Autodesk Fusion 360 part; units mm, degrees
note: some values were not read from the file. Set by a fixed rule: which sketch regions a step uses.
(part 2 of 5)
  spline S303 degree 3 poles (-4.641177, -45.308539) (-4.430839, -45.084511) (-4.24446, -44.841814) (-4.08204, -44.58107) knots 0 0 0 0 1 1 1 1
  spline S304 degree 3 poles (-4.08204, -44.58107) (-3.919308, -44.320326) (-3.783958, -44.045892) (-3.675366, -43.758389) knots 0 0 0 0 1 1 1 1
  spline S305 degree 3 poles (-3.675366, -43.758389) (-3.566775, -43.470575) (-3.487431, -43.175293) (-3.437025, -42.871922) knots 0 0 0 0 1 1 1 1
  spline S306 degree 3 poles (-3.437025, -42.871922) (-3.344302, -42.440045) (-3.20584, -42.023415) (-3.02164, -41.622031) knots 0 0 0 0 1 1 1 1
  spline S307 degree 3 poles (-3.02164, -41.622031) (-2.837439, -41.220647) (-2.611855, -40.844155) (-2.344576, -40.492244) knots 0 0 0 0 1 1 1 1
  line L5 (-2.344576, -40.492244) -> (-2.0885, -40.180472)
  spline S308 degree 3 poles (-2.0885, -40.180472) (-2.072631, -40.162736) (-2.058941, -40.143756) (-2.047117, -40.12322) knots 0 0 0 0 1 1 1 1
  spline S309 degree 3 poles (-2.047117, -40.12322) (-2.035293, -40.102684) (-2.025647, -40.081215) (-2.01818, -40.058812) knots 0 0 0 0 1 1 1 1
  spline S310 degree 3 poles (-2.01818, -40.058812) (-2.010712, -40.036409) (-2.005423, -40.013695) (-2.002622, -39.990048) knots 0 0 0 0 1 1 1 1
  spline S311 degree 3 poles (-2.002622, -39.990048) (-1.999822, -39.966711) (-1.9992, -39.943064) (-2.001067, -39.919728) knots 0 0 0 0 1 1 1 1
  spline S312 degree 3 poles (-2.001067, -39.919728) (-2.002934, -39.89608) (-2.006978, -39.872744) (-2.013513, -39.85003) knots 0 0 0 0 1 1 1 1
  spline S313 degree 3 poles (-2.013513, -39.85003) (-2.020047, -39.827316) (-2.028759, -39.805535) (-2.039649, -39.784688) knots 0 0 0 0 1 1 1 1
  spline S314 degree 3 poles (-2.039649, -39.784688) (-2.050539, -39.76353) (-2.063608, -39.743928) (-2.078232, -39.72557) knots 0 0 0 0 1 1 1 1
  spline S315 degree 3 poles (-2.078232, -39.72557) (-2.093167, -39.707212) (-2.109658, -39.690721) (-2.128016, -39.675475) knots 0 0 0 0 1 1 1 1
  spline S316 degree 3 poles (-2.128016, -39.675475) (-2.146063, -39.660539) (-2.165665, -39.647471) (-2.186512, -39.63627) knots 0 0 0 0 1 1 1 1
  spline S317 degree 3 poles (-2.186512, -39.63627) (-2.207359, -39.625379) (-2.22914, -39.616356) (-2.251854, -39.609822) knots 0 0 0 0 1 1 1 1
  spline S318 degree 3 poles (-2.251854, -39.609822) (-2.274568, -39.602979) (-2.297593, -39.598621) (-2.320929, -39.596754) knots 0 0 0 0 1 1 1 1
  spline S319 degree 3 poles (-2.320929, -39.596754) (-2.344576, -39.594578) (-2.367913, -39.594889) (-2.39156, -39.597685) knots 0 0 0 0 1 1 1 1
  spline S320 degree 3 poles (-2.39156, -39.597685) (-2.414896, -39.600169) (-2.437922, -39.605466) (-2.460324, -39.61262) knots 0 0 0 0 1 1 1 1
  spline S321 degree 3 poles (-2.460324, -39.61262) (-2.482727, -39.620083) (-2.504197, -39.629422) (-2.524732, -39.641246) knots 0 0 0 0 1 1 1 1
  spline S322 degree 3 poles (-2.524732, -39.641246) (-2.545268, -39.652758) (-2.56456, -39.666449) (-2.582295, -39.682006) knots 0 0 0 0 1 1 1 1
  spline S323 degree 3 poles (-2.582295, -39.682006) (-2.600031, -39.697564) (-2.616211, -39.714677) (-2.630524, -39.733346) knots 0 0 0 0 1 1 1 1
  line L6 (-2.630524, -39.733346) -> (-2.899669, -40.06161)
  spline S324 degree 3 poles (-2.899669, -40.06161) (-3.204285, -40.460193) (-3.460673, -40.888025) (-3.668832, -41.344482) knots 0 0 0 0 1 1 1 1
  spline S325 degree 3 poles (-3.668832, -41.344482) (-3.87668, -41.801251) (-4.031322, -42.275444) (-4.132447, -42.767061) knots 0 0 0 0 1 1 1 1
  spline S326 degree 3 poles (-12.220487, -38.608227) (-12.202752, -39.475091) (-12.270582, -40.335111) (-12.423046, -41.188596) knots 0 0 0 0 1 1 1 1
  line L7 (-12.423046, -41.188596) -> (-12.452605, -41.369997)
  spline S327 degree 3 poles (-12.452605, -41.369997) (-12.545017, -41.884328) (-12.549062, -42.399282) (-12.46474, -42.914547) knots 0 0 0 0 1 1 1 1
  spline S328 degree 3 poles (-12.46474, -42.914547) (-12.460694, -42.93695) (-12.454472, -42.95873) (-12.446071, -42.979888) knots 0 0 0 0 1 1 1 1
  spline S329 degree 3 poles (-12.446071, -42.979888) (-12.43767, -43.001047) (-12.427091, -43.021271) (-12.414956, -43.040563) knots 0 0 0 0 1 1 1 1
  spline S330 degree 3 poles (-12.414956, -43.040563) (-12.40251, -43.059543) (-12.388507, -43.077278) (-12.372951, -43.093769) knots 0 0 0 0 1 1 1 1
  spline S331 degree 3 poles (-12.372951, -43.093769) (-12.357082, -43.11026) (-12.339969, -43.124884) (-12.3213, -43.137953) knots 0 0 0 0 1 1 1 1
  spline S332 degree 3 poles (-12.3213, -43.137953) (-12.302631, -43.151021) (-12.28303, -43.162222) (-12.262181, -43.171557) knots 0 0 0 0 1 1 1 1
  spline S333 degree 3 poles (-12.262181, -43.171557) (-12.241334, -43.180891) (-12.219865, -43.188048) (-12.197773, -43.193026) knots 0 0 0 0 1 1 1 1
  spline S334 degree 3 poles (-12.197773, -43.193026) (-12.175682, -43.198005) (-12.153279, -43.201116) (-12.130565, -43.201738) knots 0 0 0 0 1 1 1 1
  spline S335 degree 3 poles (-12.130565, -43.201738) (-12.107851, -43.202375) (-12.085137, -43.201102) (-12.062734, -43.197382) knots 0 0 0 0 1 1 1 1
  spline S336 degree 3 poles (-12.062734, -43.197382) (-12.040331, -43.193646) (-12.01824, -43.187737) (-11.997081, -43.179958) knots 0 0 0 0 1 1 1 1
  spline S337 degree 3 poles (-11.997081, -43.179958) (-11.975612, -43.171868) (-11.955387, -43.161911) (-11.936096, -43.150087) knots 0 0 0 0 1 1 1 1
  spline S338 degree 3 poles (-11.936096, -43.150087) (-11.916493, -43.138264) (-11.898447, -43.124573) (-11.881645, -43.109327) knots 0 0 0 0 1 1 1 1
  spline S339 degree 3 poles (-11.881645, -43.109327) (-11.864842, -43.093769) (-11.849907, -43.076967) (-11.836217, -43.058609) knots 0 0 0 0 1 1 1 1
  spline S340 degree 3 poles (-11.836217, -43.058609) (-11.822837, -43.040251) (-11.811325, -43.02096) (-11.801368, -43.000113) knots 0 0 0 0 1 1 1 1
  spline S341 degree 3 poles (-11.801368, -43.000113) (-11.791722, -42.979577) (-11.784255, -42.958419) (-11.778654, -42.936327) knots 0 0 0 0 1 1 1 1
  spline S342 degree 3 poles (-11.778654, -42.936327) (-11.773054, -42.914236) (-11.76963, -42.891833) (-11.768386, -42.869119) knots 0 0 0 0 1 1 1 1
  spline S343 degree 3 poles (-11.768386, -42.869119) (-11.767144, -42.846405) (-11.768067, -42.823691) (-11.77119, -42.800977) knots 0 0 0 0 1 1 1 1
  spline S344 degree 3 poles (-11.77119, -42.800977) (-11.842754, -42.361633) (-11.839021, -41.9226) (-11.759677, -41.4845) knots 0 0 0 0 1 1 1 1
  line L8 (-11.759677, -41.4845) -> (-11.730429, -41.297188)
  spline S345 degree 3 poles (-11.730429, -41.297188) (-11.569563, -40.38894) (-11.500178, -39.473847) (-11.522581, -38.551909) knots 0 0 0 0 1 1 1 1
  line L9 (-11.522581, -38.551909) -> (-11.685312, -37.17538)
  spline S346 degree 3 poles (-11.685312, -37.17538) (-11.68998, -37.138042) (-11.700248, -37.102259) (-11.716116, -37.068033) knots 0 0 0 0 1 1 1 1
  spline S347 degree 3 poles (-11.716116, -37.068033) (-11.732296, -37.033806) (-11.753143, -37.003002) (-11.778969, -36.975621) knots 0 0 0 0 1 1 1 1
  spline S348 degree 3 poles (-11.778969, -36.975621) (-11.805105, -36.94824) (-11.834665, -36.925526) (-11.867646, -36.90779) knots 0 0 0 0 1 1 1 1
  spline S349 degree 3 poles (-11.867646, -36.90779) (-11.90094, -36.889744) (-11.936099, -36.877609) (-11.973126, -36.871075) knots 0 0 0 0 1 1 1 1
  spline S350 degree 3 poles (-11.973126, -36.871075) (-12.000196, -36.866096) (-12.027578, -36.864543) (-12.054959, -36.866096) knots 0 0 0 0 1 1 1 1
  spline S351 degree 3 poles (-12.054959, -36.866096) (-12.08234, -36.867338) (-12.10941, -36.872317) (-12.135547, -36.880098) knots 0 0 0 0 1 1 1 1
  spline S352 degree 3 poles (-12.135547, -36.880098) (-12.161995, -36.887879) (-12.187198, -36.898767) (-12.210845, -36.912458) knots 0 0 0 0 1 1 1 1
  spline S353 degree 3 poles (-12.210845, -36.912458) (-12.234804, -36.926148) (-12.256583, -36.942639) (-12.276809, -36.961308) knots 0 0 0 0 1 1 1 1
  spline S354 degree 3 poles (-12.276809, -36.961308) (-12.296723, -36.980288) (-12.314147, -37.001136) (-12.329393, -37.024161) knots 0 0 0 0 1 1 1 1
  spline S355 degree 3 poles (-12.329393, -37.024161) (-12.344329, -37.047186) (-12.356775, -37.071767) (-12.366109, -37.097592) knots 0 0 0 0 1 1 1 1
  spline S356 degree 3 poles (-12.366109, -37.097592) (-12.375444, -37.123418) (-12.381667, -37.150176) (-12.384778, -37.177558) knots 0 0 0 0 1 1 1 1
  spline S357 degree 3 poles (-12.384778, -37.177558) (-12.387892, -37.204939) (-12.387892, -37.23232) (-12.38446, -37.25939) knots 0 0 0 0 1 1 1 1
  line L10 (-12.38446, -37.25939) -> (-12.220487, -38.608227)
  spline S358 degree 3 poles (-10.950372, -36.928949) (-10.779861, -38.496835) (-10.819377, -40.059743) (-11.068609, -41.61705) knots 0 0 0 0 1 1 1 1
  spline S359 degree 3 poles (-11.068609, -41.61705) (-11.085722, -41.719418) (-11.097857, -41.822409) (-11.105013, -41.925711) knots 0 0 0 0 1 1 1 1
  spline S360 degree 3 poles (-11.105013, -41.925711) (-11.112166, -42.029324) (-11.114348, -42.132937) (-11.111234, -42.23655) knots 0 0 0 0 1 1 1 1
  spline S361 degree 3 poles (-11.111234, -42.23655) (-11.10812, -42.340474) (-11.100033, -42.443776) (-11.086964, -42.546456) knots 0 0 0 0 1 1 1 1
  spline S362 degree 3 poles (-11.086964, -42.546456) (-11.073896, -42.649447) (-11.055538, -42.751504) (-11.032513, -42.852628) knots 0 0 0 0 1 1 1 1
  spline S363 degree 3 poles (-11.032513, -42.852628) (-11.009488, -42.953752) (-10.981173, -43.053631) (-10.948191, -43.151954) knots 0 0 0 0 1 1 1 1
  spline S364 degree 3 poles (-10.948191, -43.151954) (-10.915209, -43.250278) (-10.87756, -43.346734) (-10.835244, -43.441324) knots 0 0 0 0 1 1 1 1
  spline S365 degree 3 poles (-10.835244, -43.441324) (-10.792927, -43.535914) (-10.745944, -43.628325) (-10.694293, -43.718248) knots 0 0 0 0 1 1 1 1
  spline S366 degree 3 poles (-10.694293, -43.718248) (-10.642953, -43.808482) (-10.586946, -43.895604) (-10.526894, -43.980236) knots 0 0 0 0 1 1 1 1
  spline S367 degree 3 poles (-10.526894, -43.980236) (-10.466842, -44.064558) (-10.403056, -44.14608) (-10.334914, -44.224178) knots 0 0 0 0 1 1 1 1
  spline S368 degree 3 poles (-10.334914, -44.224178) (-10.266773, -44.302588) (-10.195208, -44.377264) (-10.11991, -44.448206) knots 0 0 0 0 1 1 1 1
  spline S369 degree 3 poles (-10.11991, -44.448206) (-10.044301, -44.51946) (-9.96558, -44.586668) (-9.883747, -44.650143) knots 0 0 0 0 1 1 1 1
  spline S370 degree 3 poles (-9.883747, -44.650143) (-9.801604, -44.713618) (-9.716971, -44.772736) (-9.628915, -44.82781) knots 0 0 0 0 1 1 1 1
  spline S371 degree 3 poles (-9.628915, -44.82781) (-9.541171, -44.882883) (-9.450937, -44.933601) (-9.358215, -44.979651) knots 0 0 0 0 1 1 1 1
  spline S372 degree 3 poles (-9.358215, -44.979651) (-9.265492, -45.026013) (-9.170591, -45.067396) (-9.073823, -45.104422) knots 0 0 0 0 1 1 1 1
  spline S373 degree 3 poles (-9.073823, -45.104422) (-8.977055, -45.141138) (-8.878421, -45.173187) (-8.778542, -45.200257) knots 0 0 0 0 1 1 1 1
  spline S374 degree 3 poles (-8.778542, -45.200257) (-8.678662, -45.227327) (-8.577538, -45.24973) (-8.47517, -45.266843) knots 0 0 0 0 1 1 1 1
  spline S375 degree 3 poles (-8.47517, -45.266843) (-8.373113, -45.283956) (-8.270433, -45.296091) (-8.16682, -45.303247) knots 0 0 0 0 1 1 1 1
  spline S376 degree 3 poles (-8.16682, -45.303247) (-8.063518, -45.310402) (-7.960216, -45.312582) (-7.856603, -45.309468) knots 0 0 0 0 1 1 1 1
  spline S377 degree 3 poles (-7.856603, -45.309468) (-7.75299, -45.306354) (-7.649688, -45.298267) (-7.547009, -45.284887) knots 0 0 0 0 1 1 1 1
  spline S378 degree 3 poles (-7.547009, -45.284887) (-7.444329, -45.271819) (-7.342272, -45.253461) (-7.24146, -45.230125) knots 0 0 0 0 1 1 1 1
  spline S379 degree 3 poles (-7.24146, -45.230125) (-7.140336, -45.2071) (-7.040768, -45.178785) (-6.942444, -45.145803) knots 0 0 0 0 1 1 1 1
  spline S380 degree 3 poles (-6.942444, -45.145803) (-6.844121, -45.112821) (-6.747975, -45.074861) (-6.653386, -45.032544) knots 0 0 0 0 1 1 1 1
  spline S381 degree 3 poles (-6.653386, -45.032544) (-6.558796, -44.989917) (-6.466695, -44.942933) (-6.376772, -44.891282) knots 0 0 0 0 1 1 1 1
  spline S382 degree 3 poles (-6.376772, -44.891282) (-6.28685, -44.839631) (-6.199417, -44.783624) (-6.115095, -44.723572) knots 0 0 0 0 1 1 1 1
  spline S383 degree 3 poles (-6.115095, -44.723572) (-6.030773, -44.66352) (-5.949252, -44.599112) (-5.871153, -44.53097) knots 0 0 0 0 1 1 1 1
  spline S384 degree 3 poles (-5.871153, -44.53097) (-5.793055, -44.462828) (-5.718378, -44.390952) (-5.647436, -44.315654) knots 0 0 0 0 1 1 1 1
  spline S385 degree 3 poles (-5.647436, -44.315654) (-5.576183, -44.240045) (-5.508974, -44.161323) (-5.4455, -44.07918) knots 0 0 0 0 1 1 1 1
  spline S386 degree 3 poles (-5.4455, -44.07918) (-5.382336, -43.997036) (-5.322906, -43.911781) (-5.268144, -43.824037) knots 0 0 0 0 1 1 1 1
  spline S387 degree 3 poles (-5.268144, -43.824037) (-5.21307, -43.735981) (-5.162353, -43.645747) (-5.116303, -43.552714) knots 0 0 0 0 1 1 1 1
  spline S388 degree 3 poles (-5.116303, -43.552714) (-5.069941, -43.45968) (-5.028558, -43.364779) (-4.991843, -43.2677) knots 0 0 0 0 1 1 1 1
  spline S389 degree 3 poles (-4.991843, -43.2677) (-4.954816, -43.170932) (-4.922767, -43.072297) (-4.895697, -42.972107) knots 0 0 0 0 1 1 1 1
  spline S390 degree 3 poles (-4.895697, -42.972107) (-4.868627, -42.871917) (-4.846224, -42.770793) (-4.829111, -42.668424) knots 0 0 0 0 1 1 1 1
  spline S391 degree 3 poles (-4.829111, -42.668424) (-4.7423, -42.276997) (-4.627486, -41.893971) (-4.484668, -41.519346) knots 0 0 0 0 1 1 1 1
  spline S392 degree 3 poles (-4.484668, -41.519346) (-4.34185, -41.144721) (-4.172584, -40.782543) (-3.976559, -40.43281) knots 0 0 0 0 1 1 1 1
  spline S393 degree 3 poles (-3.976559, -40.43281) (-3.780846, -40.083077) (-3.560551, -39.749524) (-3.315676, -39.43215) knots 0 0 0 0 1 1 1 1
  spline S394 degree 3 poles (-3.315676, -39.43215) (-3.070801, -39.114777) (-2.804456, -38.817006) (-2.51602, -38.538838) knots 0 0 0 0 1 1 1 1
  spline S395 degree 3 poles (-2.51602, -38.538838) (-2.499529, -38.522347) (-2.485216, -38.504611) (-2.472459, -38.48532) knots 0 0 0 0 1 1 1 1
  spline S396 degree 3 poles (-2.472459, -38.48532) (-2.45939, -38.466029) (-2.448811, -38.445804) (-2.440099, -38.424334) knots 0 0 0 0 1 1 1 1
  spline S397 degree 3 poles (-2.440099, -38.424334) (-2.431076, -38.402865) (-2.424541, -38.381085) (-2.420185, -38.358371) knots 0 0 0 0 1 1 1 1
  spline S398 degree 3 poles (-2.420185, -38.358371) (-2.415518, -38.335657) (-2.41334, -38.312632) (-2.413651, -38.289606) knots 0 0 0 0 1 1 1 1
  spline S399 degree 3 poles (-2.413651, -38.289606) (-2.413651, -38.266581) (-2.415829, -38.243556) (-2.420497, -38.220842) knots 0 0 0 0 1 1 1 1
  spline S400 degree 3 poles (-2.420497, -38.220842) (-2.424853, -38.198128) (-2.431698, -38.176348) (-2.440721, -38.154878) knots 0 0 0 0 1 1 1 1
  spline S401 degree 3 poles (-2.440721, -38.154878) (-2.449434, -38.13372) (-2.460324, -38.113184) (-2.473081, -38.094204) knots 0 0 0 0 1 1 1 1
  spline S402 degree 3 poles (-2.473081, -38.094204) (-2.486149, -38.074913) (-2.500773, -38.057177) (-2.516953, -38.040997) knots 0 0 0 0 1 1 1 1
  spline S403 degree 3 poles (-2.516953, -38.040997) (-2.533444, -38.024506) (-2.55118, -38.010193) (-2.570471, -37.997125) knots 0 0 0 0 1 1 1 1
  spline S404 degree 3 poles (-2.570471, -37.997125) (-2.589762, -37.984368) (-2.609987, -37.973789) (-2.631145, -37.964766) knots 0 0 0 0 1 1 1 1
  spline S405 degree 3 poles (-2.631145, -37.964766) (-2.652615, -37.956053) (-2.674706, -37.949519) (-2.69742, -37.945163) knots 0 0 0 0 1 1 1 1
  spline S406 degree 3 poles (-2.69742, -37.945163) (-2.719823, -37.940496) (-2.742848, -37.93832) (-2.765873, -37.93832) knots 0 0 0 0 1 1 1 1
  spline S407 degree 3 poles (-2.765873, -37.93832) (-2.788898, -37.938639) (-2.811924, -37.940805) (-2.834638, -37.945474) knots 0 0 0 0 1 1 1 1
  spline S408 degree 3 poles (-2.834638, -37.945474) (-2.85704, -37.94983) (-2.879132, -37.956676) (-2.90029, -37.965699) knots 0 0 0 0 1 1 1 1
  spline S409 degree 3 poles (-2.90029, -37.965699) (-2.92176, -37.974411) (-2.941984, -37.985301) (-2.961276, -37.99837) knots 0 0 0 0 1 1 1 1
  spline S410 degree 3 poles (-2.961276, -37.99837) (-2.980256, -38.011127) (-2.997991, -38.025751) (-3.014171, -38.042242) knots 0 0 0 0 1 1 1 1
  spline S411 degree 3 poles (-3.014171, -38.042242) (-3.329367, -38.345613) (-3.620292, -38.670766) (-3.887259, -39.017698) knots 0 0 0 0 1 1 1 1
  spline S412 degree 3 poles (-3.887259, -39.017698) (-4.153915, -39.36432) (-4.393812, -39.728988) (-4.606327, -40.111391) knots 0 0 0 0 1 1 1 1
  spline S413 degree 3 poles (-4.606327, -40.111391) (-4.818843, -40.494106) (-5.00211, -40.890201) (-5.155819, -41.299985) knots 0 0 0 0 1 1 1 1
  spline S414 degree 3 poles (-5.155819, -41.299985) (-5.309216, -41.70977) (-5.431809, -42.128579) (-5.523287, -42.556721) knots 0 0 0 0 1 1 1 1
  spline S415 degree 3 poles (-5.523287, -42.556721) (-5.536666, -42.636376) (-5.55409, -42.715097) (-5.575249, -42.792885) knots 0 0 0 0 1 1 1 1
  spline S416 degree 3 poles (-5.575249, -42.792885) (-5.596407, -42.870983) (-5.621611, -42.947526) (-5.650237, -43.022825) knots 0 0 0 0 1 1 1 1
  spline S417 degree 3 poles (-5.650237, -43.022825) (-5.678862, -43.098434) (-5.711221, -43.172177) (-5.747315, -43.244364) knots 0 0 0 0 1 1 1 1
  spline S418 degree 3 poles (-5.747315, -43.244364) (-5.783408, -43.316862) (-5.822614, -43.38687) (-5.865552, -43.455323) knots 0 0 0 0 1 1 1 1
  spline S419 degree 3 poles (-5.865552, -43.455323) (-5.908491, -43.523777) (-5.954541, -43.58974) (-6.004014, -43.653837) knots 0 0 0 0 1 1 1 1
  spline S420 degree 3 poles (-6.004014, -43.653837) (-6.053487, -43.717623) (-6.105761, -43.77892) (-6.161145, -43.837416) knots 0 0 0 0 1 1 1 1
  spline S421 degree 3 poles (-6.161145, -43.837416) (-6.216529, -43.896223) (-6.274715, -43.951919) (-6.335389, -44.005126) knots 0 0 0 0 1 1 1 1
  spline S422 degree 3 poles (-6.335389, -44.005126) (-6.396374, -44.058022) (-6.459538, -44.107806) (-6.525502, -44.154478) knots 0 0 0 0 1 1 1 1
  spline S423 degree 3 poles (-6.525502, -44.154478) (-6.591154, -44.201151) (-6.658985, -44.244712) (-6.728993, -44.28485) knots 0 0 0 0 1 1 1 1
  spline S424 degree 3 poles (-6.728993, -44.28485) (-6.799002, -44.324989) (-6.870878, -44.361393) (-6.94431, -44.394375) knots 0 0 0 0 1 1 1 1
  spline S425 degree 3 poles (-6.94431, -44.394375) (-7.018053, -44.427357) (-7.09304, -44.456605) (-7.169582, -44.482431) knots 0 0 0 0 1 1 1 1
  spline S426 degree 3 poles (-7.169582, -44.482431) (-7.245815, -44.507945) (-7.323602, -44.529725) (-7.402011, -44.547772) knots 0 0 0 0 1 1 1 1
  spline S427 degree 3 poles (-7.402011, -44.547772) (-7.480732, -44.565819) (-7.560076, -44.579821) (-7.640041, -44.590089) knots 0 0 0 0 1 1 1 1
  spline S428 degree 3 poles (-7.640041, -44.590089) (-7.720007, -44.600045) (-7.800284, -44.606268) (-7.880872, -44.608758) knots 0 0 0 0 1 1 1 1
  spline S429 degree 3 poles (-7.880872, -44.608758) (-7.96146, -44.610933) (-8.041736, -44.609394) (-8.122324, -44.603779) knots 0 0 0 0 1 1 1 1
  spline S430 degree 3 poles (-8.122324, -44.603779) (-8.202601, -44.59787) (-8.282567, -44.588533) (-8.362221, -44.574842) knots 0 0 0 0 1 1 1 1
  spline S431 degree 3 poles (-8.362221, -44.574842) (-8.441565, -44.561463) (-8.520286, -44.544038) (-8.598073, -44.52288) knots 0 0 0 0 1 1 1 1
  spline S432 degree 3 poles (-8.598073, -44.52288) (-8.675861, -44.501722) (-8.752404, -44.476519) (-8.827702, -44.447893) knots 0 0 0 0 1 1 1 1
  spline S433 degree 3 poles (-8.827702, -44.447893) (-8.903, -44.418956) (-8.976743, -44.386596) (-9.048619, -44.350503) knots 0 0 0 0 1 1 1 1
  spline S434 degree 3 poles (-9.048619, -44.350503) (-9.120806, -44.314409) (-9.191126, -44.275205) (-9.259267, -44.232266) knots 0 0 0 0 1 1 1 1
  spline S435 degree 3 poles (-9.259267, -44.232266) (-9.327409, -44.189327) (-9.393373, -44.142966) (-9.457159, -44.093493) knots 0 0 0 0 1 1 1 1
  spline S436 degree 3 poles (-9.457159, -44.093493) (-9.520945, -44.04402) (-9.58193, -43.991747) (-9.640738, -43.936362) knots 0 0 0 0 1 1 1 1
  spline S437 degree 3 poles (-9.640738, -43.936362) (-9.699234, -43.880666) (-9.75493, -43.822481) (-9.807825, -43.761495) knots 0 0 0 0 1 1 1 1
  spline S438 degree 3 poles (-9.807825, -43.761495) (-9.86041, -43.700821) (-9.910194, -43.637346) (-9.956866, -43.571383) knots 0 0 0 0 1 1 1 1
  spline S439 degree 3 poles (-9.956866, -43.571383) (-10.003539, -43.50573) (-10.046789, -43.437588) (-10.086616, -43.367579) knots 0 0 0 0 1 1 1 1
  spline S440 degree 3 poles (-10.086616, -43.367579) (-10.126754, -43.29757) (-10.163159, -43.225695) (-10.19583, -43.151952) knots 0 0 0 0 1 1 1 1
  spline S441 degree 3 poles (-10.19583, -43.151952) (-10.228812, -43.078209) (-10.25806, -43.003222) (-10.283574, -42.926368) knots 0 0 0 0 1 1 1 1
  spline S442 degree 3 poles (-10.283574, -42.926368) (-10.309089, -42.849825) (-10.330869, -42.772349) (-10.348605, -42.693628) knots 0 0 0 0 1 1 1 1
  spline S443 degree 3 poles (-10.348605, -42.693628) (-10.366651, -42.614907) (-10.380653, -42.535563) (-10.39061, -42.455286) knots 0 0 0 0 1 1 1 1
  spline S444 degree 3 poles (-10.39061, -42.455286) (-10.400878, -42.375321) (-10.40679, -42.295044) (-10.408968, -42.214145) knots 0 0 0 0 1 1 1 1
  spline S445 degree 3 poles (-10.408968, -42.214145) (-10.411142, -42.133557) (-10.409605, -42.052969) (-10.403989, -41.972381) knots 0 0 0 0 1 1 1 1
  spline S446 degree 3 poles (-10.403989, -41.972381) (-10.398079, -41.891793) (-10.388432, -41.811828) (-10.375052, -41.732173) knots 0 0 0 0 1 1 1 1
  spline S447 degree 3 poles (-10.375052, -41.732173) (-10.115553, -40.106413) (-10.075104, -38.475363) (-10.254326, -36.838713) knots 0 0 0 0 1 1 1 1
  line L11 (-10.254326, -36.838713) -> (-10.390299, -35.753109)
  spline S448 degree 3 poles (-10.390299, -35.753109) (-10.394966, -35.715771) (-10.405545, -35.6803) (-10.421414, -35.646385) knots 0 0 0 0 1 1 1 1
  spline S449 degree 3 poles (-10.421414, -35.646385) (-10.437594, -35.612158) (-10.458441, -35.581665) (-10.484266, -35.554284) knots 0 0 0 0 1 1 1 1
  spline S450 degree 3 poles (-10.484266, -35.554284) (-10.510092, -35.527214) (-10.539651, -35.5045) (-10.572633, -35.486765) knots 0 0 0 0 1 1 1 1
  spline S451 degree 3 poles (-10.572633, -35.486765) (-10.605615, -35.469029) (-10.640775, -35.456894) (-10.677802, -35.45036) knots 0 0 0 0 1 1 1 1
  spline S452 degree 3 poles (-10.677802, -35.45036) (-10.71265, -35.443828) (-10.747499, -35.442897) (-10.78297, -35.447246) knots 0 0 0 0 1 1 1 1
  spline S453 degree 3 poles (-10.78297, -35.447246) (-10.805684, -35.450049) (-10.828087, -35.455027) (-10.850179, -35.462492) knots 0 0 0 0 1 1 1 1
  spline S454 degree 3 poles (-10.850179, -35.462492) (-10.871959, -35.469646) (-10.893118, -35.479295) (-10.913031, -35.490496) knots 0 0 0 0 1 1 1 1
  spline S455 degree 3 poles (-10.913031, -35.490496) (-10.932945, -35.502009) (-10.951925, -35.515388) (-10.969349, -35.530323) knots 0 0 0 0 1 1 1 1
  spline S456 degree 3 poles (-10.969349, -35.530323) (-10.986774, -35.54557) (-11.002643, -35.562372) (-11.016644, -35.580418) knots 0 0 0 0 1 1 1 1
  spline S457 degree 3 poles (-11.016644, -35.580418) (-11.030957, -35.598776) (-11.043092, -35.618379) (-11.05336, -35.638915) knots 0 0 0 0 1 1 1 1
  spline S458 degree 3 poles (-11.05336, -35.638915) (-11.063939, -35.659762) (-11.072029, -35.681231) (-11.078252, -35.703323) knots 0 0 0 0 1 1 1 1
  spline S459 degree 3 poles (-11.078252, -35.703323) (-11.084163, -35.725726) (-11.088209, -35.74844) (-11.089765, -35.771465) knots 0 0 0 0 1 1 1 1
  spline S460 degree 3 poles (-11.089765, -35.771465) (-11.091318, -35.79449) (-11.091007, -35.817515) (-11.0879, -35.84054) knots 0 0 0 0 1 1 1 1
  line L12 (-11.0879, -35.84054) -> (-10.950372, -36.928949)
  spline S461 degree 3 poles (-9.684301, -41.864103) (-9.694258, -41.921044) (-9.701414, -41.977984) (-9.705459, -42.035547) knots 0 0 0 0 1 1 1 1
  spline S462 degree 3 poles (-9.705459, -42.035547) (-9.709817, -42.09311) (-9.71137, -42.150673) (-9.710127, -42.208236) knots 0 0 0 0 1 1 1 1
  spline S463 degree 3 poles (-9.710127, -42.208236) (-9.708573, -42.265798) (-9.704527, -42.323361) (-9.69737, -42.380302) knots 0 0 0 0 1 1 1 1
  spline S464 degree 3 poles (-9.69737, -42.380302) (-9.690527, -42.437553) (-9.680567, -42.494494) (-9.668121, -42.550501) knots 0 0 0 0 1 1 1 1
  spline S465 degree 3 poles (-9.668121, -42.550501) (-9.655675, -42.606819) (-9.640118, -42.662204) (-9.622382, -42.716966) knots 0 0 0 0 1 1 1 1
  spline S466 degree 3 poles (-9.622382, -42.716966) (-9.604336, -42.771729) (-9.583489, -42.825558) (-9.560152, -42.878142) knots 0 0 0 0 1 1 1 1
  spline S467 degree 3 poles (-9.560152, -42.878142) (-9.537127, -42.931038) (-9.511302, -42.982377) (-9.482987, -43.032473) knots 0 0 0 0 1 1 1 1
  spline S468 degree 3 poles (-9.482987, -43.032473) (-9.454672, -43.082568) (-9.423868, -43.131418) (-9.390575, -43.178402) knots 0 0 0 0 1 1 1 1
  spline S469 degree 3 poles (-9.390575, -43.178402) (-9.357593, -43.225697) (-9.322433, -43.271125) (-9.284784, -43.314686) knots 0 0 0 0 1 1 1 1
  spline S470 degree 3 poles (-9.284784, -43.314686) (-9.247135, -43.358247) (-9.207619, -43.399941) (-9.165925, -43.439768) knots 0 0 0 0 1 1 1 1
  spline S471 degree 3 poles (-9.165925, -43.439768) (-9.124231, -43.479596) (-9.08067, -43.517245) (-9.035242, -43.552716) knots 0 0 0 0 1 1 1 1
  spline S472 degree 3 poles (-9.035242, -43.552716) (-8.990125, -43.588187) (-8.943141, -43.62148) (-8.894291, -43.652284) knots 0 0 0 0 1 1 1 1
  spline S473 degree 3 poles (-8.894291, -43.652284) (-8.845751, -43.683088) (-8.795967, -43.711403) (-8.744316, -43.737228) knots 0 0 0 0 1 1 1 1
  spline S474 degree 3 poles (-8.744316, -43.737228) (-8.692976, -43.763365) (-8.640392, -43.786701) (-8.586874, -43.807548) knots 0 0 0 0 1 1 1 1
  spline S475 degree 3 poles (-8.586874, -43.807548) (-8.533045, -43.828084) (-8.478594, -43.846131) (-8.423209, -43.861688) knots 0 0 0 0 1 1 1 1
  spline S476 degree 3 poles (-8.423209, -43.861688) (-8.367514, -43.876935) (-8.311506, -43.889692) (-8.254877, -43.899649) knots 0 0 0 0 1 1 1 1
  spline S477 degree 3 poles (-8.254877, -43.899649) (-8.198247, -43.909294) (-8.140996, -43.916451) (-8.083744, -43.920807) knots 0 0 0 0 1 1 1 1
  spline S478 degree 3 poles (-8.083744, -43.920807) (-8.026181, -43.925163) (-7.968619, -43.926407) (-7.911056, -43.925163) knots 0 0 0 0 1 1 1 1
  spline S479 degree 3 poles (-7.911056, -43.925163) (-7.853804, -43.92361) (-7.796241, -43.919562) (-7.739301, -43.912406) knots 0 0 0 0 1 1 1 1
  spline S480 degree 3 poles (-7.739301, -43.912406) (-7.682049, -43.905244) (-7.62542, -43.895604) (-7.569102, -43.882846) knots 0 0 0 0 1 1 1 1
  spline S481 degree 3 poles (-7.569102, -43.882846) (-7.513095, -43.8704) (-7.45771, -43.855154) (-7.402947, -43.837107) knots 0 0 0 0 1 1 1 1
  spline S482 degree 3 poles (-7.402947, -43.837107) (-7.348185, -43.818749) (-7.294668, -43.798214) (-7.242083, -43.774877) knots 0 0 0 0 1 1 1 1
  spline S483 degree 3 poles (-7.242083, -43.774877) (-7.189187, -43.751541) (-7.137847, -43.725716) (-7.087752, -43.697401) knots 0 0 0 0 1 1 1 1
  spline S484 degree 3 poles (-7.087752, -43.697401) (-7.037657, -43.668775) (-6.989117, -43.637971) (-6.942134, -43.604989) knots 0 0 0 0 1 1 1 1
  spline S485 degree 3 poles (-6.942134, -43.604989) (-6.894839, -43.571696) (-6.849723, -43.536225) (-6.805851, -43.498576) knots 0 0 0 0 1 1 1 1
  spline S486 degree 3 poles (-6.805851, -43.498576) (-6.762289, -43.460927) (-6.720595, -43.421411) (-6.681079, -43.379716) knots 0 0 0 0 1 1 1 1
  spline S487 degree 3 poles (-6.681079, -43.379716) (-6.641252, -43.338022) (-6.603603, -43.294461) (-6.568132, -43.249033) knots 0 0 0 0 1 1 1 1
  spline S488 degree 3 poles (-6.568132, -43.249033) (-6.532661, -43.203605) (-6.499679, -43.15631) (-6.468564, -43.107771) knots 0 0 0 0 1 1 1 1
  spline S489 degree 3 poles (-6.468564, -43.107771) (-6.43776, -43.05892) (-6.409446, -43.009136) (-6.38362, -42.957485) knots 0 0 0 0 1 1 1 1
  spline S490 degree 3 poles (-6.38362, -42.957485) (-6.357795, -42.906146) (-6.334147, -42.853561) (-6.313611, -42.799732) knots 0 0 0 0 1 1 1 1
  spline S491 degree 3 poles (-6.313611, -42.799732) (-6.292764, -42.745903) (-6.274718, -42.691141) (-6.25916, -42.635756) knots 0 0 0 0 1 1 1 1
  spline S492 degree 3 poles (-6.25916, -42.635756) (-6.243914, -42.58006) (-6.231156, -42.524053) (-6.221511, -42.467113) knots 0 0 0 0 1 1 1 1
  spline S493 degree 3 poles (-6.221511, -42.467113) (-6.11043, -41.954337) (-5.959522, -41.453385) (-5.768476, -40.964568) knots 0 0 0 0 1 1 1 1
  spline S494 degree 3 poles (-5.768476, -40.964568) (-5.57743, -40.475751) (-5.348734, -40.005292) (-5.08239, -39.55319) knots 0 0 0 0 1 1 1 1
  spline S495 degree 3 poles (-5.08239, -39.55319) (-4.816045, -39.101089) (-4.515474, -38.673257) (-4.180676, -38.269384) knots 0 0 0 0 1 1 1 1
  spline S496 degree 3 poles (-4.180676, -38.269384) (-3.845878, -37.865511) (-3.48121, -37.490886) (-3.086361, -37.145509) knots 0 0 0 0 1 1 1 1
  spline S497 degree 3 poles (-3.086361, -37.145509) (-3.06987, -37.129952) (-3.054934, -37.112527) (-3.041555, -37.094169) knots 0 0 0 0 1 1 1 1
  spline S498 degree 3 poles (-3.041555, -37.094169) (-3.028175, -37.0755) (-3.016974, -37.055587) (-3.007328, -37.035051) knots 0 0 0 0 1 1 1 1
  spline S499 degree 3 poles (-3.007328, -37.035051) (-2.997994, -37.014204) (-2.990526, -36.992423) (-2.985237, -36.970332) knots 0 0 0 0 1 1 1 1
  spline S500 degree 3 poles (-2.985237, -36.970332) (-2.979947, -36.947929) (-2.976836, -36.925526) (-2.976213, -36.902501) knots 0 0 0 0 1 1 1 1
  spline S501 degree 3 poles (-2.976213, -36.902501) (-2.97528, -36.879787) (-2.976524, -36.857073) (-2.980258, -36.834359) knots 0 0 0 0 1 1 1 1
  spline S502 degree 3 poles (-2.980258, -36.834359) (-2.983681, -36.811956) (-2.989282, -36.789864) (-2.997372, -36.768395) knots 0 0 0 0 1 1 1 1
  spline S503 degree 3 poles (-2.997372, -36.768395) (-3.00515, -36.746926) (-3.014796, -36.72639) (-3.02662, -36.706787) knots 0 0 0 0 1 1 1 1
  spline S504 degree 3 poles (-3.02662, -36.706787) (-3.038443, -36.687185) (-3.052134, -36.669138) (-3.067692, -36.652336) knots 0 0 0 0 1 1 1 1
  spline S505 degree 3 poles (-3.067692, -36.652336) (-3.082938, -36.635223) (-3.09974, -36.619976) (-3.118098, -36.606286) knots 0 0 0 0 1 1 1 1
  spline S506 degree 3 poles (-3.118098, -36.606286) (-3.136456, -36.592906) (-3.156058, -36.581083) (-3.176594, -36.571437) knots 0 0 0 0 1 1 1 1
  spline S507 degree 3 poles (-3.176594, -36.571437) (-3.19713, -36.56148) (-3.218599, -36.553701) (-3.240691, -36.548101) knots 0 0 0 0 1 1 1 1
  spline S508 degree 3 poles (-3.240691, -36.548101) (-3.262783, -36.5425) (-3.285497, -36.539077) (-3.308211, -36.537833) knots 0 0 0 0 1 1 1 1
  spline S509 degree 3 poles (-3.308211, -36.537833) (-3.330925, -36.536591) (-3.353639, -36.537514) (-3.376353, -36.540947) knots 0 0 0 0 1 1 1 1
  spline S510 degree 3 poles (-3.376353, -36.540947) (-3.399067, -36.544061) (-3.421158, -36.549348) (-3.442628, -36.556815) knots 0 0 0 0 1 1 1 1
  spline S511 degree 3 poles (-3.442628, -36.556815) (-3.464097, -36.564278) (-3.484944, -36.573929) (-3.504547, -36.585441) knots 0 0 0 0 1 1 1 1
  spline S512 degree 3 poles (-3.504547, -36.585441) (-3.524149, -36.596954) (-3.542818, -36.610333) (-3.559931, -36.62558) knots 0 0 0 0 1 1 1 1
  spline S513 degree 3 poles (-3.559931, -36.62558) (-3.985585, -36.99616) (-4.378568, -37.398788) (-4.73888, -37.833465) knots 0 0 0 0 1 1 1 1
  spline S514 degree 3 poles (-4.73888, -37.833465) (-5.099192, -38.268142) (-5.422166, -38.729267) (-5.707179, -39.216528) knots 0 0 0 0 1 1 1 1
  spline S515 degree 3 poles (-5.707179, -39.216528) (-5.992504, -39.703789) (-6.236757, -40.210964) (-6.439316, -40.738053) knots 0 0 0 0 1 1 1 1
  spline S516 degree 3 poles (-6.439316, -40.738053) (-6.642185, -41.265141) (-6.801183, -41.805298) (-6.915998, -42.358212) knots 0 0 0 0 1 1 1 1
  spline S517 degree 3 poles (-6.915998, -42.358212) (-6.928444, -42.426354) (-6.947424, -42.492941) (-6.972938, -42.557349) knots 0 0 0 0 1 1 1 1
  spline S518 degree 3 poles (-6.972938, -42.557349) (-6.998453, -42.621757) (-7.029879, -42.683364) (-7.067528, -42.74155) knots 0 0 0 0 1 1 1 1
  spline S519 degree 3 poles (-7.067528, -42.74155) (-7.105177, -42.799735) (-7.147805, -42.853875) (-7.196034, -42.903659) knots 0 0 0 0 1 1 1 1
  spline S520 degree 3 poles (-7.196034, -42.903659) (-7.244261, -42.953443) (-7.296846, -42.998249) (-7.353786, -43.037765) knots 0 0 0 0 1 1 1 1
  spline S521 degree 3 poles (-7.353786, -43.037765) (-7.410727, -43.07697) (-7.47109, -43.110574) (-7.534564, -43.138266) knots 0 0 0 0 1 1 1 1
  spline S522 degree 3 poles (-7.534564, -43.138266) (-7.598351, -43.165647) (-7.664002, -43.186806) (-7.731522, -43.20143) knots 0 0 0 0 1 1 1 1
  spline S523 degree 3 poles (-7.731522, -43.20143) (-7.799353, -43.216054) (-7.867806, -43.223833) (-7.937192, -43.225077) knots 0 0 0 0 1 1 1 1
  spline S524 degree 3 poles (-7.937192, -43.225077) (-8.006268, -43.226319) (-8.075032, -43.22041) (-8.143174, -43.207964) knots 0 0 0 0 1 1 1 1
  spline S525 degree 3 poles (-8.143174, -43.207964) (-8.211316, -43.195518) (-8.277591, -43.176538) (-8.341999, -43.151023) knots 0 0 0 0 1 1 1 1
  spline S526 degree 3 poles (-8.341999, -43.151023) (-8.406407, -43.125509) (-8.467704, -43.094083) (-8.525889, -43.056434) knots 0 0 0 0 1 1 1 1
  spline S527 degree 3 poles (-8.525889, -43.056434) (-8.584074, -43.018785) (-8.637903, -42.975846) (-8.687687, -42.927617) knots 0 0 0 0 1 1 1 1
  spline S528 degree 3 poles (-8.687687, -42.927617) (-8.737471, -42.879389) (-8.781965, -42.826805) (-8.82117, -42.769553) knots 0 0 0 0 1 1 1 1
  spline S529 degree 3 poles (-8.82117, -42.769553) (-8.860686, -42.712613) (-8.893979, -42.652249) (-8.921672, -42.588464) knots 0 0 0 0 1 1 1 1
  spline S530 degree 3 poles (-8.921672, -42.588464) (-8.949053, -42.524989) (-8.9699, -42.459336) (-8.984524, -42.391506) knots 0 0 0 0 1 1 1 1
  spline S531 degree 3 poles (-8.984524, -42.391506) (-8.999148, -42.323675) (-9.006927, -42.254911) (-9.00786, -42.185835) knots 0 0 0 0 1 1 1 1
  spline S532 degree 3 poles (-9.00786, -42.185835) (-9.009103, -42.116449) (-9.003193, -42.047684) (-8.990747, -41.979231) knots 0 0 0 0 1 1 1 1
  spline S533 degree 3 poles (-8.990747, -41.979231) (-8.85353, -41.313059) (-8.663729, -40.661821) (-8.421342, -40.026141) knots 0 0 0 0 1 1 1 1
  spline S534 degree 3 poles (-8.421342, -40.026141) (-8.178956, -39.390461) (-7.887408, -38.778117) (-7.546388, -38.189421) knots 0 0 0 0 1 1 1 1
  spline S535 degree 3 poles (-7.546388, -38.189421) (-7.205367, -37.601036) (-6.819541, -37.043454) (-6.388598, -36.517299) knots 0 0 0 0 1 1 1 1
  spline S536 degree 3 poles (-6.388598, -36.517299) (-5.957654, -35.990833) (-5.487507, -35.502638) (-4.977842, -35.052404) knots 0 0 0 0 1 1 1 1
  spline S537 degree 3 poles (-4.977842, -35.052404) (-4.961351, -35.036535) (-4.946416, -35.019422) (-4.933036, -35.000753) knots 0 0 0 0 1 1 1 1
  spline S538 degree 3 poles (-4.933036, -35.000753) (-4.919657, -34.982084) (-4.908455, -34.962481) (-4.899121, -34.941634) knots 0 0 0 0 1 1 1 1
  spline S539 degree 3 poles (-4.899121, -34.941634) (-4.889475, -34.920787) (-4.882319, -34.899318) (-4.877029, -34.876915) knots 0 0 0 0 1 1 1 1
  spline S540 degree 3 poles (-4.877029, -34.876915) (-4.87174, -34.854823) (-4.868628, -34.832109) (-4.867695, -34.809395) knots 0 0 0 0 1 1 1 1
  spline S541 degree 3 poles (-4.867695, -34.809395) (-4.866761, -34.786681) (-4.868316, -34.763967) (-4.87174, -34.741253) knots 0 0 0 0 1 1 1 1
  spline S542 degree 3 poles (-4.87174, -34.741253) (-4.875162, -34.718539) (-4.881074, -34.696759) (-4.888853, -34.67529) knots 0 0 0 0 1 1 1 1
  spline S543 degree 3 poles (-4.888853, -34.67529) (-4.896632, -34.65382) (-4.906589, -34.633284) (-4.918412, -34.613682) knots 0 0 0 0 1 1 1 1
  spline S544 degree 3 poles (-4.918412, -34.613682) (-4.930236, -34.594079) (-4.943927, -34.575721) (-4.959173, -34.558919) knots 0 0 0 0 1 1 1 1
  spline S545 degree 3 poles (-4.959173, -34.558919) (-4.974419, -34.542117) (-4.991533, -34.526871) (-5.00989, -34.51318) knots 0 0 0 0 1 1 1 1
  spline S546 degree 3 poles (-5.00989, -34.51318) (-5.028248, -34.49949) (-5.04754, -34.487977) (-5.068387, -34.47802) knots 0 0 0 0 1 1 1 1
  spline S547 degree 3 poles (-5.068387, -34.47802) (-5.088923, -34.468375) (-5.110392, -34.460596) (-5.132484, -34.454995) knots 0 0 0 0 1 1 1 1
  spline S548 degree 3 poles (-5.132484, -34.454995) (-5.154575, -34.449394) (-5.176979, -34.445972) (-5.199693, -34.444727) knots 0 0 0 0 1 1 1 1
  spline S549 degree 3 poles (-5.199693, -34.444727) (-5.222718, -34.443485) (-5.245431, -34.444409) (-5.267834, -34.44753) knots 0 0 0 0 1 1 1 1
  spline S550 degree 3 poles (-5.267834, -34.44753) (-5.290548, -34.450955) (-5.31264, -34.456242) (-5.33411, -34.46371) knots 0 0 0 0 1 1 1 1
  spline S551 degree 3 poles (-5.33411, -34.46371) (-5.35589, -34.471173) (-5.376426, -34.480823) (-5.396029, -34.492336) knots 0 0 0 0 1 1 1 1
  spline S552 degree 3 poles (-5.396029, -34.492336) (-5.415942, -34.503848) (-5.4343, -34.517228) (-5.451413, -34.532163) knots 0 0 0 0 1 1 1 1
  spline S553 degree 3 poles (-5.451413, -34.532163) (-5.990014, -35.008845) (-6.486611, -35.525977) (-6.941823, -36.082936) knots 0 0 0 0 1 1 1 1
  spline S554 degree 3 poles (-6.941823, -36.082936) (-7.396725, -36.640206) (-7.804331, -37.230147) (-8.164021, -37.853381) knots 0 0 0 0 1 1 1 1
  spline S555 degree 3 poles (-8.164021, -37.853381) (-8.523711, -38.476304) (-8.831127, -39.12443) (-9.08627, -39.797137) knots 0 0 0 0 1 1 1 1
  spline S556 degree 3 poles (-9.08627, -39.797137) (-9.341102, -40.470155) (-9.54055, -41.159042) (-9.684301, -41.864103) knots 0 0 0 0 1 1 1 1
  spline S557 degree 3 poles (-7.477001, -40.476062) (-7.495048, -40.469841) (-7.513095, -40.465172) (-7.531764, -40.46206) knots 0 0 0 0 1 1 1 1
  spline S558 degree 3 poles (-7.531764, -40.46206) (-7.572835, -40.454597) (-7.613907, -40.454597) (-7.654979, -40.46206) knots 0 0 0 0 1 1 1 1
  spline S559 degree 3 poles (-7.654979, -40.46206) (-7.696051, -40.469523) (-7.734634, -40.483841) (-7.770727, -40.504999) knots 0 0 0 0 1 1 1 1
  spline S560 degree 3 poles (-7.770727, -40.504999) (-7.80682, -40.526157) (-7.837935, -40.552916) (-7.864383, -40.585276) knots 0 0 0 0 1 1 1 1
  spline S561 degree 3 poles (-7.864383, -40.585276) (-7.891142, -40.617324) (-7.911056, -40.653418) (-7.925057, -40.692934) knots 0 0 0 0 1 1 1 1
  spline S562 degree 3 poles (-7.925057, -40.692934) (-8.095257, -41.159348) (-8.22065, -41.637586) (-8.300927, -42.127336) knots 0 0 0 0 1 1 1 1
  spline S563 degree 3 poles (-8.300927, -42.127336) (-8.304352, -42.150362) (-8.305594, -42.173387) (-8.304352, -42.196723) knots 0 0 0 0 1 1 1 1
  spline S564 degree 3 poles (-8.304352, -42.196723) (-8.30311, -42.219748) (-8.299685, -42.242462) (-8.293773, -42.265176) knots 0 0 0 0 1 1 1 1
  spline S565 degree 3 poles (-8.293773, -42.265176) (-8.288174, -42.287579) (-8.280082, -42.309048) (-8.269814, -42.329895) knots 0 0 0 0 1 1 1 1
  spline S566 degree 3 poles (-8.269814, -42.329895) (-8.259858, -42.350742) (-8.247723, -42.370345) (-8.233721, -42.389014) knots 0 0 0 0 1 1 1 1
  spline S567 degree 3 poles (-8.233721, -42.389014) (-8.219719, -42.407372) (-8.203851, -42.424174) (-8.186426, -42.43942) knots 0 0 0 0 1 1 1 1
  spline S568 degree 3 poles (-8.186426, -42.43942) (-8.169002, -42.454667) (-8.150333, -42.468046) (-8.130108, -42.479559) knots 0 0 0 0 1 1 1 1
  spline S569 degree 3 poles (-8.130108, -42.479559) (-8.109883, -42.491071) (-8.089036, -42.500406) (-8.066944, -42.507562) knots 0 0 0 0 1 1 1 1
  spline S570 degree 3 poles (-8.066944, -42.507562) (-8.044853, -42.514716) (-8.02245, -42.519697) (-7.999425, -42.522497) knots 0 0 0 0 1 1 1 1
  spline S571 degree 3 poles (-7.999425, -42.522497) (-7.9764, -42.5253) (-7.953686, -42.526234) (-7.930661, -42.524673) knots 0 0 0 0 1 1 1 1
  spline S572 degree 3 poles (-7.930661, -42.524673) (-7.907636, -42.52312) (-7.884922, -42.519383) (-7.86283, -42.513472) knots 0 0 0 0 1 1 1 1
  spline S573 degree 3 poles (-7.86283, -42.513472) (-7.840427, -42.507562) (-7.818958, -42.49947) (-7.798111, -42.489202) knots 0 0 0 0 1 1 1 1
  spline S574 degree 3 poles (-7.798111, -42.489202) (-7.777575, -42.479245) (-7.757972, -42.46711) (-7.739614, -42.453108) knots 0 0 0 0 1 1 1 1
  spline S575 degree 3 poles (-7.739614, -42.453108) (-7.721568, -42.439107) (-7.704766, -42.423238) (-7.689519, -42.406125) knots 0 0 0 0 1 1 1 1
  spline S576 degree 3 poles (-7.689519, -42.406125) (-7.674273, -42.3887) (-7.660893, -42.370031) (-7.64907, -42.350118) knots 0 0 0 0 1 1 1 1
  spline S577 degree 3 poles (-7.64907, -42.350118) (-7.637557, -42.330204) (-7.628224, -42.309046) (-7.620756, -42.287265) knots 0 0 0 0 1 1 1 1
  spline S578 degree 3 poles (-7.620756, -42.287265) (-7.613292, -42.265485) (-7.607999, -42.243082) (-7.604887, -42.220368) knots 0 0 0 0 1 1 1 1
  spline S579 degree 3 poles (-7.604887, -42.220368) (-7.528967, -41.777601) (-7.414152, -41.345102) (-7.260444, -40.922871) knots 0 0 0 0 1 1 1 1
  spline S580 degree 3 poles (-7.260444, -40.922871) (-7.252981, -40.901091) (-7.247687, -40.878688) (-7.244575, -40.855974) knots 0 0 0 0 1 1 1 1
  spline S581 degree 3 poles (-7.244575, -40.855974) (-7.241461, -40.83326) (-7.240529, -40.810235) (-7.241771, -40.78721) knots 0 0 0 0 1 1 1 1
  spline S582 degree 3 poles (-7.241771, -40.78721) (-7.243325, -40.764185) (-7.24675, -40.741471) (-7.252662, -40.719068) knots 0 0 0 0 1 1 1 1
  spline S583 degree 3 poles (-7.252662, -40.719068) (-7.258572, -40.696976) (-7.266353, -40.675507) (-7.27662, -40.65466) knots 0 0 0 0 1 1 1 1
  spline S584 degree 3 poles (-7.27662, -40.65466) (-7.286577, -40.633813) (-7.298401, -40.61421) (-7.312403, -40.595852) knots 0 0 0 0 1 1 1 1
  spline S585 degree 3 poles (-7.312403, -40.595852) (-7.326404, -40.577494) (-7.341962, -40.560692) (-7.359075, -40.545446) knots 0 0 0 0 1 1 1 1
  spline S586 degree 3 poles (-7.359075, -40.545446) (-7.376188, -40.529888) (-7.394857, -40.516509) (-7.414771, -40.504996) knots 0 0 0 0 1 1 1 1
  spline S587 degree 3 poles (-7.414771, -40.504996) (-7.434373, -40.493173) (-7.455221, -40.483527) (-7.477001, -40.476062) knots 0 0 0 0 1 1 1 1
  spline S588 degree 3 poles (-7.182031, -39.783441) (-7.161495, -39.793709) (-7.140025, -39.80211) (-7.117622, -39.808022) knots 0 0 0 0 1 1 1 1
  spline S589 degree 3 poles (-7.117622, -39.808022) (-7.095531, -39.814243) (-7.072817, -39.817979) (-7.049792, -39.819535) knots 0 0 0 0 1 1 1 1
  spline S590 degree 3 poles (-7.049792, -39.819535) (-7.026767, -39.821399) (-7.003741, -39.820777) (-6.981028, -39.81767) knots 0 0 0 0 1 1 1 1
  spline S591 degree 3 poles (-6.981028, -39.81767) (-6.958002, -39.814868) (-6.935599, -39.809889) (-6.913819, -39.802424) knots 0 0 0 0 1 1 1 1
  spline S592 degree 3 poles (-6.913819, -39.802424) (-6.891727, -39.79527) (-6.87088, -39.785622) (-6.850656, -39.77442) knots 0 0 0 0 1 1 1 1
  spline S593 degree 3 poles (-6.850656, -39.77442) (-6.830742, -39.762908) (-6.812072, -39.749528) (-6.794648, -39.734282) knots 0 0 0 0 1 1 1 1
  spline S594 degree 3 poles (-6.794648, -39.734282) (-6.777223, -39.719347) (-6.761355, -39.702545) (-6.747043, -39.684187) knots 0 0 0 0 1 1 1 1
  spline S595 degree 3 poles (-6.747043, -39.684187) (-6.733041, -39.66614) (-6.720905, -39.646538) (-6.710327, -39.626002) knots 0 0 0 0 1 1 1 1
  spline S596 degree 3 poles (-6.710327, -39.626002) (-6.357171, -38.924669) (-5.939296, -38.263786) (-5.457636, -37.643974) knots 0 0 0 0 1 1 1 1
  spline S597 degree 3 poles (-5.457636, -37.643974) (-4.975975, -37.023852) (-4.43893, -36.456003) (-3.846811, -35.940738) knots 0 0 0 0 1 1 1 1
  spline S598 degree 3 poles (-3.846811, -35.940738) (-3.829386, -35.925491) (-3.813829, -35.908689) (-3.799827, -35.890331) knots 0 0 0 0 1 1 1 1
  spline S599 degree 3 poles (-3.799827, -35.890331) (-3.785514, -35.871974) (-3.773379, -35.852371) (-3.763111, -35.831835) knots 0 0 0 0 1 1 1 1
  spline S600 degree 3 poles (-3.763111, -35.831835) (-3.753154, -35.810988) (-3.745065, -35.789519) (-3.738842, -35.767116) knots 0 0 0 0 1 1 1 1
  spline S601 degree 3 poles (-3.738842, -35.767116) (-3.73293, -35.744713) (-3.729196, -35.721999) (-3.72764, -35.698974) knots 0 0 0 0 1 1 1 1
  spline S602 degree 3 poles (-3.72764, -35.698974) (-3.726084, -35.675949) (-3.727019, -35.652924) (-3.729818, -35.63021) knots 0 0 0 0 1 1 1 1
  spline S603 degree 3 poles (-3.729818, -35.63021) (-3.73293, -35.607185) (-3.737908, -35.584782) (-3.745376, -35.563001) knots 0 0 0 0 1 1 1 1
  spline S604 degree 3 poles (-3.745376, -35.563001) (-3.752843, -35.54091) (-3.762178, -35.520063) (-3.77369, -35.500149) knots 0 0 0 0 1 1 1 1
  spline S605 degree 3 poles (-3.77369, -35.500149) (-3.785514, -35.479924) (-3.798582, -35.461255) (-3.813829, -35.443831) knots 0 0 0 0 1 1 1 1
  spline S606 degree 3 poles (-3.813829, -35.443831) (-3.829075, -35.426406) (-3.845877, -35.410849) (-3.864235, -35.396847) knots 0 0 0 0 1 1 1 1
  spline S607 degree 3 poles (-3.864235, -35.396847) (-3.882593, -35.382534) (-3.901884, -35.370399) (-3.922731, -35.360131) knots 0 0 0 0 1 1 1 1
  spline S608 degree 3 poles (-3.922731, -35.360131) (-3.943267, -35.349863) (-3.964737, -35.341773) (-3.987139, -35.335862) knots 0 0 0 0 1 1 1 1
  spline S609 degree 3 poles (-3.987139, -35.335862) (-4.009542, -35.329952) (-4.032256, -35.326216) (-4.055281, -35.32466) knots 0 0 0 0 1 1 1 1
  spline S610 degree 3 poles (-4.055281, -35.32466) (-4.078306, -35.323107) (-4.10102, -35.323729) (-4.124046, -35.326836) knots 0 0 0 0 1 1 1 1
  spline S611 degree 3 poles (-4.124046, -35.326836) (-4.14676, -35.32995) (-4.169162, -35.334926) (-4.191254, -35.342393) knots 0 0 0 0 1 1 1 1
  spline S612 degree 3 poles (-4.191254, -35.342393) (-4.213035, -35.349856) (-4.233882, -35.359195) (-4.254106, -35.371019) knots 0 0 0 0 1 1 1 1
  spline S613 degree 3 poles (-4.254106, -35.371019) (-4.27402, -35.382532) (-4.292689, -35.395911) (-4.310113, -35.411158) knots 0 0 0 0 1 1 1 1
  spline S614 degree 3 poles (-4.310113, -35.411158) (-4.936459, -35.956604) (-5.504308, -36.557435) (-6.013972, -37.213651) knots 0 0 0 0 1 1 1 1
  spline S615 degree 3 poles (-6.013972, -37.213651) (-6.523637, -37.869867) (-6.96547, -38.569022) (-7.339162, -39.311426) knots 0 0 0 0 1 1 1 1
  spline S616 degree 3 poles (-7.339162, -39.311426) (-7.349429, -39.331962) (-7.357831, -39.353432) (-7.363742, -39.375835) knots 0 0 0 0 1 1 1 1
  spline S617 degree 3 poles (-7.363742, -39.375835) (-7.369964, -39.397926) (-7.373699, -39.42064) (-7.375256, -39.443665) knots 0 0 0 0 1 1 1 1
  spline S618 degree 3 poles (-7.375256, -39.443665) (-7.377119, -39.46669) (-7.376498, -39.489716) (-7.373392, -39.512741) knots 0 0 0 0 1 1 1 1
  spline S619 degree 3 poles (-7.373392, -39.512741) (-7.370588, -39.535766) (-7.365609, -39.558169) (-7.358145, -39.579949) knots 0 0 0 0 1 1 1 1
  spline S620 degree 3 poles (-7.358145, -39.579949) (-7.350993, -39.602041) (-7.341654, -39.622888) (-7.330142, -39.643113) knots 0 0 0 0 1 1 1 1
  spline S621 degree 3 poles (-7.330142, -39.643113) (-7.318629, -39.663026) (-7.305561, -39.681695) (-7.290315, -39.699431) knots 0 0 0 0 1 1 1 1
  spline S622 degree 3 poles (-7.290315, -39.699431) (-7.275379, -39.716855) (-7.258577, -39.732413) (-7.240219, -39.746726) knots 0 0 0 0 1 1 1 1
  spline S623 degree 3 poles (-7.240219, -39.746726) (-7.222173, -39.761039) (-7.202571, -39.773173) (-7.182031, -39.783441) knots 0 0 0 0 1 1 1 1
  spline S624 degree 3 poles (-9.614915, -36.433597) (-9.537438, -36.960375) (-9.476764, -37.515467) (-9.476142, -37.516089) knots 0 0 0 0 1 1 1 1
  spline S625 degree 3 poles (-9.476142, -37.516089) (-9.472096, -37.552183) (-9.462763, -37.58672) (-9.448138, -37.619702) knots 0 0 0 0 1 1 1 1
  spline S626 degree 3 poles (-9.448138, -37.619702) (-9.433514, -37.652684) (-9.414223, -37.682866) (-9.390264, -37.709936) knots 0 0 0 0 1 1 1 1
  spline S627 degree 3 poles (-9.390264, -37.709936) (-9.366306, -37.737317) (-9.338924, -37.760031) (-9.307809, -37.7787) knots 0 0 0 0 1 1 1 1
  spline S628 degree 3 poles (-9.307809, -37.7787) (-9.277005, -37.797369) (-9.243712, -37.810749) (-9.208552, -37.819461) knots 0 0 0 0 1 1 1 1
  spline S629 degree 3 poles (-9.208552, -37.819461) (-9.173392, -37.827862) (-9.137921, -37.830662) (-9.101828, -37.828173) knots 0 0 0 0 1 1 1 1
  spline S630 degree 3 poles (-9.101828, -37.828173) (-9.065734, -37.82537) (-9.030886, -37.817594) (-8.997281, -37.804214) knots 0 0 0 0 1 1 1 1
  spline S631 degree 3 poles (-8.997281, -37.804214) (-8.963677, -37.790835) (-8.932873, -37.772788) (-8.90487, -37.750074) knots 0 0 0 0 1 1 1 1
  spline S632 degree 3 poles (-8.90487, -37.750074) (-8.876866, -37.727049) (-8.852908, -37.700601) (-8.832994, -37.670109) knots 0 0 0 0 1 1 1 1
  spline S633 degree 3 poles (-8.832994, -37.670109) (-8.154998, -36.642379) (-7.409481, -35.66599) (-6.596445, -34.741251) knots 0 0 0 0 1 1 1 1
  spline S634 degree 3 poles (-6.596445, -34.741251) (-6.580888, -34.724138) (-6.566886, -34.70578) (-6.555062, -34.686177) knots 0 0 0 0 1 1 1 1
  spline S635 degree 3 poles (-6.555062, -34.686177) (-6.542927, -34.666264) (-6.53297, -34.645728) (-6.525192, -34.623947) knots 0 0 0 0 1 1 1 1
  spline S636 degree 3 poles (-6.525192, -34.623947) (-6.517102, -34.602167) (-6.511502, -34.580075) (-6.508078, -34.55705) knots 0 0 0 0 1 1 1 1
  spline S637 degree 3 poles (-6.508078, -34.55705) (-6.504343, -34.534336) (-6.5031, -34.511311) (-6.504032, -34.488286) knots 0 0 0 0 1 1 1 1
  spline S638 degree 3 poles (-6.504032, -34.488286) (-6.505275, -34.465261) (-6.50839, -34.442236) (-6.513678, -34.419833) knots 0 0 0 0 1 1 1 1